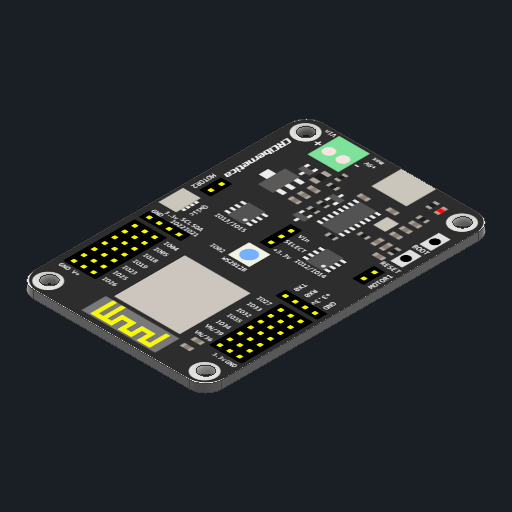
# Autodesk Inventor part: ideaboard
Saved by Autodesk Inventor 2026.2 (Build 302298000, 298)
## iProperties
Created: 2025-06-04
Part Number: ideaboard
Material: Generic
Document SubType Name: Modeling
Designer: cdavi
Density: 1 g/cm^3
Appearance: Default
Mass: 6.66356 g
Surface Area: 72.1379 cm^2
Volume: 6.66356 cm^3
Finish3_Appearance: Smooth - Black
Finish3_Process: Prime/Paint RAL 3018
Finish3_Description: Prime/Paint RAL 3018
Finish3_ShortDescription: RAL 3018
Finish3_Thickness: 0,050 mm
Finish3_Area: 128,000 mm^2
Author: cdavi
Autodesk Inventor part; units mm, degrees
ref_plane "YZ Plane" through (0, 0, 0) normal (1, 0, 0) x (0, 1, 0)
ref_plane "XZ Plane" through (0, 0, 0) normal (0, 1, 0) x (-1, 0, 0)
ref_plane "XY Plane" through (0, 0, 0) normal (0, 0, 1) x (1, 0, 0)
sketch "Sketch1" plane through (0, 0, 0) normal (0, 1, 0) x (-1, 0, 0)
  line L0 (-23.5, 36) -> (-23.5, -36)
  line L1 (-23.5, -36) -> (23.5, -36)
  line L2 (23.5, -36) -> (23.5, 36)
  line L3 (23.5, 36) -> (-23.5, 36)
  line L4 (-23.5, 36) -> (23.5, -36) construction
  line L5 (-23.5, -36) -> (23.5, 36) construction
  point P0 (0, 0)
  dimension "d0" = 72
  dimension "d1" = 47
  constraints: 12 end point, 2 midpoint, 2 parallel, 1 perpendicular, 1 vertical
  measures "d0" distance of L1.end L2.end
  measures "d1" distance of L2.end L0.start
extrude "Extrusion1" add sketch "Sketch1" along normal blind 2
sketch "Sketch3" plane through (0, 2, 0) normal (0, 1, 0) x (1, 0, 0)
  line L0 (-23.5, 36) -> (-23.5, -36) projected
  line L1 (23.5, -36) -> (23.5, 36) projected
  line L2 (-23.535, 36.3293) -> (23.5, 36.3293) construction
  line L3 (23.5, 36.3293) -> (23.5, -36) construction
  line L4 (23.5, -36) -> (-23.535, -36) construction
  line L5 (-23.535, -36) -> (-23.535, 36.3293) construction
  point P0 (0, 0)
  constraints: 1 coincident, 1 vertical, 2 other
sketch "Sketch4" plane through (0, 2, 0) normal (0, 1, 0) x (1, 0, 0)
  line L0 (-23.5, 36) -> (-23.5, -36) projected
  line L1 (-23.5, -36) -> (23.5, -36) projected
  line L2 (23.5, -36) -> (23.5, 36) projected
  line L3 (23.5, 36) -> (-23.5, 36) projected
  point P0 (0, 0)
fillet "Fillet1" radius 4 4 edges at (23.5, 1, 36) (-23.5, 1, 36) (23.5, 1, -36) (-23.5, 1, -36)
decal "Decal1"
sketch "Sketch5" plane through (0, 2, 0) normal (0, 1, 0) x (1, 0, 0)
  line L0 (-19.5, 32) -> (-19.5, -32)
  line L1 (-19.5, -32) -> (19.5, -32)
  line L2 (19.5, -32) -> (19.5, 32)
  line L3 (19.5, 32) -> (-19.5, 32)
  line L4 (-19.5, 32) -> (19.5, -32) construction
  line L5 (-19.5, -32) -> (19.5, 32) construction
  circle A0 centre (-19.5, 32) radius 1.75
  line L6 (0, 32) -> (0, -32)
  line L7 (19.5, 0) -> (-19.5, 0)
  circle A1 centre (19.5, 32) radius 1.75
  circle A2 centre (-19.5, -32) radius 1.75
  circle A3 centre (19.5, -32) radius 1.75
  point P0 (0, 0)
  dimension "d37" = 39
  dimension "d38" = 64
  dimension "d39" = 3.5
  constraints: 16 end point, 6 midpoint, 4 centre point, 3 symmetric about line, 2 parallel, 1 coincident, 1 perpendicular, 1 vertical, 3 other
  measures "d37" distance between parallel lines of L0 L2
  measures "d38" distance of L1.end L2.end
  measures "d39" diameter of A0
extrude "Extrusion2" cut sketch "Sketch5" against normal through all contours L3 A0 L0 | L0 A0 L3 | A2 L1 L0 | L0 L1 A2 | A1 L2 L3 | L3 L2 A1 | A3 L2 L1 | L1 L2 A3
body "Solid1"
